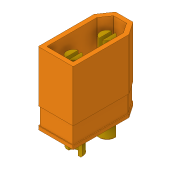
# Autodesk Inventor part: stecker1
Saved by Autodesk Inventor 2017 (Build 210142000, 142)
## iProperties
Part Number: stecker1
Material: Generisch
Document SubType Name: Modeling
Designer: ExCISS
Density: 1 g/cm^3
Appearance: Vorgabe
Author: ExCISS
Autodesk Inventor part; units mm, degrees
ref_plane "YZ Plane" through (0, 0, 0) normal (1, 0, 0) x (0, 1, 0)
ref_plane "XZ Plane" through (0, 0, 0) normal (0, 1, 0) x (-1, 0, 0)
ref_plane "XY Plane" through (0, 0, 0) normal (0, 0, 1) x (1, 0, 0)
sketch "Skizze1" plane through (0, 0, 0) normal (0, 0, 1) x (1, 0, 0)
  line L0 (-2.6, -5.1) -> (2.6, -5.1)
  line L1 (2.6, -5.1) -> (2.6, 3.2)
  line L2 (-2.6, -5.1) -> (-2.6, 3.2)
  line L3 (-1.3, 5.1) -> (1.3, 5.1)
  line L4 (0, -5.1) -> (0, 5.1) construction
  line L5 (-2.6, 3.2) -> (-1.3, 5.1)
  line L6 (1.3, 5.1) -> (2.6, 3.2)
  point P0 (0, 0)
  point P1 (0, 0)
  point P2 (0, 0)
  dimension "d0" = 5.2
  dimension "d1" = 8.3
  dimension "d2" = 2.6
  dimension "d3" = 10.2
  constraints: 14 end point, 3 midpoint, 2 horizontal, 2 vertical, 1 coincident, 1 parallel, 1 perpendicular
  measures "d0" distance of L0.start L0.end
  measures "d1" distance of L0.end L1.end
  measures "d2" distance of L3.start L3.end
  measures "d3" distance of L4.end L4.start
extrude "Extrusion1" add sketch "Skizze1" along normal blind 10.7
shell "Wandung1" thickness 0.63 removed faces 1 at (-0.8667, 0.4333, 10.7)
sketch "Skizze2" plane through (-1.97, -4.47, 0.63) normal (0, 0, 1) x (1, 0, 0)
  line L0 (1.9995, 1.9801) -> (1.9995, 6.9801) construction
  circle A0 centre (1.9995, 6.9801) radius 1
  circle A1 centre (1.9995, 1.9801) radius 1
  point P0 (1.97, 4.47)
  point P1 (0, 0)
  point P2 (1.9995, 4.4801)
  point P3 (1.9995, 4.4801)
  dimension "d7" = 5
  dimension "d8" = 2
  dimension "d9" = 2
  constraints: 3 coincident, 2 centre point, 2 end point, 1 midpoint, 1 vertical
  measures "d7" distance of L0.start L0.end
  measures "d8" diameter of A0
  measures "d9" diameter of A1
extrude "Extrusion2" add sketch "Skizze2" along normal blind 9
sketch "Skizze3" plane through (2.6, -5.1, 0) normal (1, 0, 0) x (0, 0, -1)
  line L0 (0, 0) -> (-10.7, 0) projected
  line L1 (0, 8.3) -> (-10.7, 8.3) construction
  line L2 (0, 0) -> (-0.52, 0)
  line L3 (-0.52, 0) -> (-0.52, 8.3) construction
  line L4 (-0.52, 8.3) -> (0, 8.3)
  line L5 (0, 8.3) -> (0, 0) construction
  line L6 (-0.52, 0) -> (-3.07, 0)
  line L7 (-3.07, 0) -> (-3.07, 8.3)
  line L8 (-3.07, 8.3) -> (-0.52, 8.3)
  line L9 (-0.52, 8.3) -> (-0.52, 0)
  point P0 (0, 5.1)
  dimension "d12" = 0.52
  dimension "d13" = 2.55
  constraints: 16 end point, 4 parallel, 2 horizontal, 2 perpendicular, 2 point on line
  measures "d12" distance of L3.end L4.end
  measures "d13" distance of L7.end L8.end
extrude "Extrusion3" cut sketch "Skizze3" against normal blind 0.1
sketch "Skizze4" plane through (-2.6, -5.1, 0) normal (0, -1, 0) x (1, 0, 0)
  line L0 (0, 0) -> (0, 10.7) construction
  line L1 (5.2, 0.52) -> (5.2, 3.07) construction
  line L2 (0, 0) -> (5.2, 0) construction
  line L3 (5.2, 0) -> (5.2, 0.52) construction
  line L4 (5.2, 0.52) -> (0, 0.52) construction
  line L5 (0, 0.52) -> (0, 0) construction
  line L6 (5.2, 3.07) -> (5.2, 10.7) projected
  line L7 (0, 0.52) -> (5.2, 0.52)
  line L8 (5.2, 0.52) -> (5.2, 3.07)
  line L9 (5.2, 3.07) -> (0, 3.07)
  line L10 (0, 3.07) -> (0, 0.52)
  point P0 (2.6, 0)
  dimension "d16" = 0.52
  dimension "d17" = 2.55
  constraints: 16 end point, 4 parallel, 2 horizontal, 2 perpendicular
  measures "d16" distance of L1.start L2.end
  measures "d17" distance of L1.end L7.end
extrude "Extrusion4" cut sketch "Skizze4" against normal blind 0.1
sketch "Skizze5" plane through (1.3, 5.1, 10.7) normal (0.8253073, 0.5646839, 0) x (0, 0, -1)
  line L0 (10.7, -2.3022) -> (10.18, -2.3022) construction
  line L1 (10.7, 0) -> (0, 0) construction
  line L2 (10.18, -2.3022) -> (10.7, -2.3022) construction
  line L3 (10.7, -2.3022) -> (10.7, 0) construction
  line L4 (10.7, 0) -> (10.18, 0) construction
  line L5 (10.18, 0) -> (10.18, -2.3022) construction
  line L6 (10.18, -2.3022) -> (7.63, -2.3022)
  line L7 (7.63, -2.3022) -> (7.63, 0)
  line L8 (7.63, 0) -> (10.18, 0)
  line L9 (10.18, 0) -> (10.18, -2.3022)
  point P0 (10.7, -3.475)
  dimension "d20" = 2.55
  constraints: 16 end point, 4 parallel, 2 horizontal, 2 perpendicular, 1 point on line
  measures "d20" distance of L7.end L8.end
extrude "Extrusion5" cut sketch "Skizze5" against normal blind 0.1
sketch "Skizze6" plane through (-1.3, 5.1, 0) normal (0, 1, 0) x (1, 0, 0)
  line L0 (-1.3, 0) -> (3.9, 0) construction
  line L1 (3.8, -0.52) -> (-1.3, -0.52) construction
  line L2 (2.6079, 0) -> (-0.0061, 0) construction
  line L3 (-0.0061, 0) -> (-0.0061, -0.52) construction
  line L4 (-0.0061, -0.52) -> (2.6079, -0.52) construction
  line L5 (2.6079, -0.52) -> (2.6079, 0) construction
  line L6 (2.6, -0.52) -> (2.6, -3.07) projected
  line L7 (-1.3, -3.07) -> (3.8, -3.07) projected
  line L8 (2.6, -0.52) -> (-0.0061, -0.52)
  line L9 (-0.0061, -0.52) -> (-0.0061, -3.07)
  line L10 (-0.0061, -3.07) -> (2.6, -3.07)
  line L11 (2.6, -3.07) -> (2.6, -0.52)
  point P0 (1.3, 0)
  constraints: 16 end point, 4 parallel, 4 point on line, 2 horizontal, 2 perpendicular
extrude "Extrusion6" cut sketch "Skizze6" against normal blind 0.1
sketch "Skizze7" plane through (-2.6, 3.2, 0) normal (-0.8253073, 0.5646839, 0) x (0, 0, 1)
  line L0 (0, 2.3022) -> (0.52, 2.3022) construction
  line L1 (0, 0) -> (10.7, 0) construction
  line L2 (0.52, 2.3022) -> (0, 2.3022) construction
  line L3 (0, 2.3022) -> (0, 0) construction
  line L4 (0, 0) -> (0.52, 0) construction
  line L5 (0.52, 0) -> (0.52, 2.3022) construction
  line L6 (0, 2.3022) -> (0, 0) construction
  line L7 (0.52, -3.9137) -> (0.52, -6.8501) construction
  line L8 (0, 0) -> (0.52, 0) construction
  line L9 (0.52, 0) -> (0.52, -6.8501) construction
  line L10 (0.52, -6.8501) -> (0, -6.8501) construction
  line L11 (0, -6.8501) -> (0, 0) construction
  line L12 (3.07, -3.8876) -> (3.07, 2.8544) projected
  line L13 (0.52, 2.3022) -> (3.07, 2.3022)
  line L14 (3.07, 2.3022) -> (3.07, 0)
  line L15 (3.07, 0) -> (0.52, 0)
  line L16 (0.52, 0) -> (0.52, 2.3022)
  line L17 (3.07, 0) -> (0.52, 0)
  line L18 (0.52, 0) -> (0.52, -6.8501)
  line L19 (0.52, -6.8501) -> (3.07, -6.8501)
  line L20 (3.07, -6.8501) -> (3.07, 0)
  point P0 (0, -1.1728)
  constraints: 32 end point, 8 parallel, 4 horizontal, 4 perpendicular, 2 point on line
extrude "Extrusion7" cut sketch "Skizze7" against normal blind 0.1
sketch "Skizze8" plane through (-2.6, -5.1, 0) normal (-1, 0, 0) x (0, 0, 1)
  line L0 (0.52, 10.2) -> (0.52, 8.3) projected
  line L1 (0, 0) -> (0.52, 0) construction
  line L2 (0.52, 8.3) -> (0, 8.3) construction
  line L3 (0, 8.3) -> (0, 0) construction
  line L4 (0, 0) -> (0.52, 0) construction
  line L5 (0.52, 0) -> (0.52, 8.3) construction
  line L6 (3.07, 0) -> (10.7, 0) projected
  line L7 (0.52, 8.3) -> (3.07, 8.3)
  line L8 (3.07, 8.3) -> (3.07, 0)
  line L9 (3.07, 0) -> (0.52, 0)
  line L10 (0.52, 0) -> (0.52, 8.3)
  point P0 (0, 5.1)
  constraints: 16 end point, 4 parallel, 2 horizontal, 2 perpendicular
extrude "Extrusion8" cut sketch "Skizze8" against normal blind 0.1
fillet "Rundung1" radius 0.1 22 edges at (-2.5, 3.1655, 1.795) (-2.5, -5, 1.795) (-2.6, -5.1, 6.885) (-2.6, 3.2, 6.885) (2.5, -5, 1.795) (2.6, -5.1, 6.885) (-2.6, -5.1, 0.26) (2.6, -5.1, 0.26) (-2.6, 3.2, 0.26) (-1.3, 5.1, 0.26) (-1.2448, 5, 1.795) (-1.3, 5.1, 6.885) (1.3, 5.1, 6.885) (1.2448, 5, 1.795) (1.3, 5.1, 0.26) (2.6, 3.2, 0.26) (2.5, 3.1655, 1.795) (2.6, 3.2, 6.885) (-1.97, 3.0051, 5.665) (-0.9677, 4.47, 5.665) (1.97, 3.0051, 5.665) (0.9677, 4.47, 5.665)
fillet "Rundung2" radius 0.1 1 edges at (-1.97, -4.47, 5.665)
fillet "Rundung3" radius 0.1 1 edges at (1.97, -4.47, 5.665)
sketch "Skizze9" plane through (0.0295, 2.5101, 9.63) normal (0, 0, 1) x (1, 0, 0)
  circle A0 centre (0, 0) radius 1 construction
  line L0 (-0.25, 1) -> (0.25, 1)
  line L1 (0.25, 1) -> (0.25, -1)
  line L2 (0.25, -1) -> (-0.25, -1)
  line L3 (-0.25, -1) -> (-0.25, 1)
  line L4 (-0.25, 1) -> (0.25, -1) construction
  point P0 (-0.0295, -2.5101)
  dimension "d34" = 0.5
  dimension "d35" = 2
  constraints: 10 end point, 2 parallel, 1 coincident, 1 horizontal, 1 midpoint, 1 perpendicular
  measures "d34" distance of L1.end L2.end
  measures "d35" distance of L0.end L1.end
extrude "Extrusion9" cut sketch "Skizze9" against normal blind 7
sketch "Skizze10" plane through (0.0295, -2.4899, 9.63) normal (0, 0, 1) x (1, 0, 0)
  circle A0 centre (0, 0) radius 1 projected
  line L0 (-0.25, 1) -> (0.25, 1)
  line L1 (0.25, 1) -> (0.25, -1)
  line L2 (0.25, -1) -> (-0.25, -1)
  line L3 (-0.25, -1) -> (-0.25, 1)
  line L4 (-0.25, 1) -> (0.25, -1) construction
  point P0 (-0.0295, 2.4899)
  dimension "d38" = 0.5
  dimension "d39" = 2
  constraints: 10 end point, 2 parallel, 1 coincident, 1 horizontal, 1 midpoint, 1 perpendicular
  measures "d38" distance of L1.end L2.end
  measures "d39" distance of L0.end L1.end
extrude "Extrusion10" cut sketch "Skizze10" against normal blind 7 contours L1 A0 L3 | A0 L0 L1 | L1 L2 A0 | A0 L3 L0 | L2 L3 A0
sketch "Skizze11" plane through (0, 0, 0) normal (0, 0, -1) x (-1, 0, 0)
  arc A0 (-1.97, -4.37) -> (-1.87, -4.47) centre (-1.87, -4.37) ccw construction
  line L0 (-1.97, -4.37) -> (-1.97, 2.9742) construction
  arc A1 (-1.9525, 3.0306) -> (-1.97, 2.9742) centre (-1.87, 2.9742) ccw construction
  line L1 (-1.9525, 3.0306) -> (-0.9975, 4.4265) construction
  arc A2 (-0.915, 4.47) -> (-0.9975, 4.4265) centre (-0.915, 4.37) ccw construction
  line L2 (-0.915, 4.47) -> (0.915, 4.47) construction
  arc A3 (0.9975, 4.4265) -> (0.915, 4.47) centre (0.915, 4.37) ccw construction
  line L3 (0.9975, 4.4265) -> (1.9525, 3.0306) construction
  arc A4 (1.97, 2.9742) -> (1.9525, 3.0306) centre (1.87, 2.9742) ccw construction
  line L4 (1.97, 2.9742) -> (1.97, -4.37) construction
  arc A5 (1.87, -4.47) -> (1.97, -4.37) centre (1.87, -4.37) ccw construction
  line L5 (1.87, -4.47) -> (-1.87, -4.47) construction
  circle A6 centre (-0.0295, 2.5101) radius 1 construction
  circle A7 centre (-0.0295, -2.4899) radius 1 construction
  circle A8 centre (-0.0295, -2.4899) radius 1.3
  circle A9 centre (-0.0295, 2.5101) radius 1.3
  point P0 (0, 0)
  dimension "d42" = 2.6
  constraints: 2 centre point, 2 coincident, 1 equal radius
  measures "d42" diameter of A9
extrude "Extrusion11" add sketch "Skizze11" along normal blind 3
chamfer "Fase1" distance 0.2 angle 45 2 edges at (1.3295, -2.4899, -3) (1.3295, 2.5101, -3)
sketch "Skizze12" plane through (0.0295, -2.4899, -3) normal (0, 0, -1) x (-1, 0, 0)
  circle A0 centre (0, 0) radius 1.1 projected
  circle A1 centre (0, 5) radius 1.1 projected
  point P0 (0.0295, 2.4899)
hole "Bohrung1" at (0.0295, 2.5101, -3) at (0.0295, -2.4899, -3) direction (0, 0, 1) diameter 1.4 depth 4.5 tip angle 118
sketch "Skizze13" plane through (0.0295, -2.4899, -3) normal (0, 0, -1) x (-1, 0, 0)
  circle A0 centre (0, 0) radius 1.3 construction
  circle A1 centre (0, 5) radius 1.3 construction
  arc A2 (-2.553, 5.7155) -> (-2.5705, 5.659) centre (-2.4705, 5.659) ccw construction
  line L0 (-2.5705, -2.5101) -> (-2.5705, 5.659) construction
  arc A3 (-2.5705, -2.5101) -> (-2.4705, -2.6101) centre (-2.4705, -2.5101) ccw construction
  line L1 (2.5295, -2.6101) -> (-2.4705, -2.6101) construction
  arc A4 (2.5295, -2.6101) -> (2.6295, -2.5101) centre (2.5295, -2.5101) ccw construction
  line L2 (2.6295, 5.659) -> (2.6295, -2.5101) construction
  arc A5 (2.6295, 5.659) -> (2.612, 5.7155) centre (2.5295, 5.659) ccw construction
  line L3 (1.3593, 7.5464) -> (2.612, 5.7155) construction
  arc A6 (1.3593, 7.5464) -> (1.2767, 7.5899) centre (1.2767, 7.4899) ccw construction
  line L4 (-1.2178, 7.5899) -> (1.2767, 7.5899) construction
  arc A7 (-1.2178, 7.5899) -> (-1.3003, 7.5464) centre (-1.2178, 7.4899) ccw construction
  line L5 (-2.553, 5.7155) -> (-1.3003, 7.5464) construction
  line L6 (-1.3, 0) -> (1.3, 0)
  line L7 (-1.3, 5) -> (1.3, 5)
  arc A8 (-1.3, 0) -> (1.3, 0) centre (0, 0) ccw
  arc A9 (1.3, 5) -> (-1.3, 5) centre (0, 5) ccw
  point P0 (0.0295, 2.4899)
  constraints: 4 coincident, 4 end point, 4 point on circle, 2 centre point, 2 horizontal, 2 horizontal alignment, 2 midpoint, 2 other
extrude "Extrusion12" cut sketch "Skizze13" against normal blind 2.5
